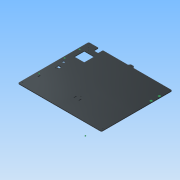
# Autodesk Inventor part: боковая  панель
Saved by Autodesk Inventor 2017 (Build 210142000, 142)
## iProperties
Part Number: боковая  панель
Material: Типовые
Document SubType Name: Modeling
Designer: Max
Mass: 347.039 g
Surface Area: 2371.89 cm^2
Volume: 347.039 cm^3
Density: 1 g/cm^3
Appearance: Чугун серый
Author: Max
Autodesk Inventor part; units mm, degrees
ref_plane "YZ Plane" through (0, 0, 0) normal (1, 0, 0) x (0, 1, 0)
ref_plane "XZ Plane" through (0, 0, 0) normal (0, 1, 0) x (-1, 0, 0)
ref_plane "XY Plane" through (0, 0, 0) normal (0, 0, 1) x (1, 0, 0)
sketch "Эскиз1" plane through (0, 0, 0) normal (0, 0, 1) x (1, 0, 0)
  circle A0 centre (10.6994, 67.6713) radius 1.5
  circle A1 centre (10.6994, 364.6713) radius 1.5
  circle A2 centre (-348.3006, 364.6713) radius 1.5
  circle A3 centre (-348.3006, 67.6713) radius 1.5
  line L0 (-355.8006, 370.6713) -> (18.1994, 370.6713)
  line L1 (18.1994, 370.6713) -> (18.1994, 53.6713)
  line L2 (18.1994, 53.6713) -> (-355.8006, 53.6713)
  line L3 (-355.8006, 53.6713) -> (-355.8006, 370.6713)
  point P0 (18.1994, 53.6713)
  dimension "d4" = 374
  dimension "d6" = 317
  dimension "d7" = 14
  dimension "d40" = 7.5
  dimension "d41" = 297
  dimension "d42" = 7.5
  dimension "d43" = 7.5
  dimension "d44" = 297
  dimension "d45" = 6
  dimension "d46" = 359
  dimension "d47" = 14
  dimension "d48" = 359
  constraints: 8 end point, 4 centre point, 2 parallel, 1 coincident, 1 horizontal, 1 perpendicular
  measures "d4" distance between parallel lines of L1 L3
  measures "d6" distance between parallel lines of L0 L2
  measures "d7" distance from line of A3.centre L2
  measures "d40" distance from line of L1 A0.centre
  measures "d41" distance of A0.centre A1.centre
  measures "d42" distance from line of L1 A1.centre
  measures "d43" distance from line of L3 A2.centre
  measures "d44" distance of A3.centre A2.centre
  measures "d45" distance from line of L0 A2.centre
  measures "d46" distance of A0.centre A3.centre
  measures "d47" distance from line of L2 A0.centre
  measures "d48" distance of A1.centre A2.centre
extrude "Выдавливание1" add sketch "Эскиз1" along normal blind 3
sketch "Эскиз3" plane through (0, 0, 3) normal (0, 0, 1) x (1, 0, 0)
  circle A0 centre (10.6994, 282.6713) radius 3.75 projected
  circle A1 centre (10.6994, 319.6713) radius 3.75 projected
  circle A2 centre (-348.3006, 321.6713) radius 2 projected
  circle A3 centre (-348.3006, 254.6713) radius 2 projected
  circle A4 centre (-345.3006, 137.6713) radius 1.5 projected
  point P0 (0, 0)
sketch "Эскиз4" plane through (0, 0, 3) normal (0, 0, 1) x (1, 0, 0)
  circle A0 centre (-168.3006, 372.6713) radius 1.5 projected
  line L0 (-179.3006, 370.6713) -> (-175.8006, 378.6713)
  line L1 (-175.8006, 378.6713) -> (-160.8006, 378.6713)
  line L2 (-160.8006, 378.6713) -> (-157.3006, 370.6713)
  line L3 (18.1994, 370.6713) -> (-355.8006, 370.6713) projected
  line L4 (-168.3006, 372.6713) -> (-168.3006, 378.6713)
  point P0 (0, 0)
  dimension "d49" = 8
  dimension "d50" = 22
  dimension "d51" = 15
  constraints: 8 end point, 2 point on line, 1 horizontal, 1 midpoint, 1 perpendicular, 1 other
  measures "d49" distance between parallel lines of L3 L1
  measures "d50" distance of L0.start L2.end
  measures "d51" distance of L0.end L1.end
extrude "Выдавливание3" add sketch "Эскиз4" against normal blind 3
fillet "Сопряжение1" radius 5 4 edges at (-179.3006, 370.6713, 1.5) (-157.3006, 370.6713, 1.5) (-160.8006, 378.6713, 1.5) (-175.8006, 378.6713, 1.5)
fillet "Сопряжение2" radius 5 4 edges at (-355.8006, 370.6713, 1.5) (18.1994, 370.6713, 1.5) (18.1994, 53.6713, 1.5) (-355.8006, 53.6713, 1.5)
sketch "Эскиз5" plane through (0, 0, 3) normal (0, 0, 1) x (1, 0, 0)
  line L0 (-332.3006, 327.1713) -> (-287.3006, 327.1713)
  line L1 (-287.3006, 327.1713) -> (-287.3006, 282.1713)
  line L2 (-287.3006, 282.1713) -> (-332.3006, 282.1713)
  line L3 (-332.3006, 282.1713) -> (-332.3006, 327.1713)
  line L4 (-355.8006, 365.6713) -> (-355.8006, 58.6713) projected
  line L5 (-182.5707, 370.6713) -> (-350.8006, 370.6713) projected
  line L6 (-312.3006, 370.6713) -> (-292.3006, 370.6713)
  line L7 (-292.3006, 370.6713) -> (-292.3006, 349.1713)
  line L8 (-292.3006, 349.1713) -> (-312.3006, 349.1713)
  line L9 (-312.3006, 349.1713) -> (-312.3006, 370.6713)
  circle A0 centre (-335.8006, 238.6713) radius 4.95
  line L10 (-333.3006, 213.1713) -> (-320.3006, 213.1713)
  line L11 (-320.3006, 213.1713) -> (-320.3006, 203.1713)
  line L12 (-320.3006, 203.1713) -> (-333.3006, 203.1713)
  line L13 (-333.3006, 203.1713) -> (-333.3006, 213.1713)
  circle A1 centre (-330.4506, 196.6713) radius 1.6
  circle A2 centre (-323.1506, 196.6713) radius 1.6
  line L14 (-330.4506, 196.6713) -> (-323.1506, 196.6713)
  line L15 (-326.8006, 203.1713) -> (-326.8006, 196.6713)
  circle A3 centre (-162.8006, 142.6713) radius 1.6
  line L16 (18.1994, 58.6713) -> (18.1994, 365.6713) projected
  line L17 (-350.8006, 53.6713) -> (13.1994, 53.6713) projected
  line L18 (-173.8006, 132.1713) -> (-173.8006, 123.1713) construction
  line L19 (-175.3006, 132.1713) -> (-175.3006, 123.1713)
  line L20 (-172.3006, 123.1713) -> (-172.3006, 132.1713)
  arc A4 (-172.3006, 132.1713) -> (-175.3006, 132.1713) centre (-173.8006, 132.1713) ccw
  arc A5 (-175.3006, 123.1713) -> (-172.3006, 123.1713) centre (-173.8006, 123.1713) ccw
  line L21 (-151.8006, 132.1713) -> (-151.8006, 123.1713) construction
  line L22 (-153.3006, 132.1713) -> (-153.3006, 123.1713)
  line L23 (-150.3006, 123.1713) -> (-150.3006, 132.1713)
  arc A6 (-150.3006, 132.1713) -> (-153.3006, 132.1713) centre (-151.8006, 132.1713) ccw
  arc A7 (-153.3006, 123.1713) -> (-150.3006, 123.1713) centre (-151.8006, 123.1713) ccw
  line L24 (-162.8006, 142.6713) -> (-162.8006, 102.5696) construction
  line L25 (-173.8006, 127.6713) -> (-151.8006, 127.6713) construction
  circle A8 centre (-346.3006, 134.6713) radius 1.6
  line L26 (-335.3006, 132.1713) -> (-335.3006, 123.1713)
  line L27 (-336.8006, 132.1713) -> (-336.8006, 123.1713)
  line L28 (-333.8006, 123.1713) -> (-333.8006, 132.1713)
  arc A9 (-333.8006, 132.1713) -> (-336.8006, 132.1713) centre (-335.3006, 132.1713) ccw
  arc A10 (-336.8006, 123.1713) -> (-333.8006, 123.1713) centre (-335.3006, 123.1713) ccw
  circle A11 centre (-334.3006, 349.1713) radius 1.45
  circle A12 centre (-325.3006, 338.6713) radius 1.45
  circle A13 centre (10.6994, 319.6713) radius 3.75 construction
  circle A14 centre (10.6994, 282.6713) radius 3.75 construction
  circle A15 centre (10.6994, 319.6713) radius 4.75
  circle A16 centre (10.6994, 282.6713) radius 4.75
  point P0 (0, 0)
  point P1 (-335.3006, 127.6713)
  dimension "d56" = 68.5
  dimension "d57" = 45
  dimension "d58" = 45
  dimension "d59" = 23.5
  dimension "d60" = 43.5
  dimension "d61" = 21.5
  dimension "d62" = 20
  dimension "d63" = 43.5
  dimension "d64" = 20
  dimension "d65" = 132
  dimension "d66" = 9.9
  dimension "d67" = 13
  dimension "d68" = 10
  dimension "d69" = 157.5
  dimension "d70" = 22.5
  dimension "d71" = 3.2
  dimension "d72" = 3.2
  dimension "d73" = 10.5
  dimension "d74" = 6.5
  dimension "d75" = 7.3
  dimension "d76" = 193
  dimension "d77" = 181
  dimension "d78" = 89
  dimension "d79" = 3.2
  dimension "d80" = 22
  dimension "d81" = 12
  dimension "d82" = 3
  dimension "d83" = 3
  dimension "d84" = 12
  dimension "d85" = 25
  dimension "d86" = 68
  dimension "d87" = 3.2
  dimension "d88" = 9.5
  dimension "d89" = 81
  dimension "d90" = 3
  dimension "d91" = 68
  dimension "d92" = 19
  dimension "d93" = 12
  dimension "d94" = 2.9
  dimension "d95" = 2.9
  dimension "d96" = 21.5
  dimension "d97" = 21.5
  dimension "d98" = 32
  dimension "d99" = 30.5
  dimension "d100" = 9.5
  dimension "d101" = 9.5
  constraints: 56 end point, 15 centre point, 12 point on circle, 12 tangent, 10 parallel, 5 horizontal, 5 midpoint, 4 perpendicular, 3 coincident, 3 vertical, 1 point on line, 1 symmetric about line, 1 other
  measures "d56" distance between parallel lines of L1 L4
  measures "d57" distance between parallel lines of L2 L0
  measures "d58" distance between parallel lines of L1 L3
  measures "d59" distance between parallel lines of L3 L4
  measures "d60" distance between parallel lines of L0 L5
  measures "d61" distance between parallel lines of L8 L5
  measures "d62" distance between parallel lines of L7 L9
  measures "d63" distance between parallel lines of L9 L4
  measures "d64" distance from line of L4 A0.centre
  measures "d65" distance from line of L5 A0.centre
  measures "d66" diameter of A0
  measures "d67" distance of L11.end L12.end
  measures "d68" distance of L10.end L11.end
  measures "d69" distance between parallel lines of L5 L10
  measures "d70" distance between parallel lines of L4 L13
  measures "d71" diameter of A2
  measures "d72" diameter of A1
  measures "d74" distance from line of L12 L14.start
  measures "d75" distance of L14.end L14.start
  measures "d76" distance from line of L4 L24.start
  measures "d77" distance from line of L16 L24.start
  measures "d78" distance from line of L17 L24.start
  measures "d79" diameter of A3
  measures "d80" distance between parallel lines of L21 L18
  measures "d82" distance between parallel lines of L20 L19
  measures "d83" distance between parallel lines of L23 L22
  measures "d85" distance between parallel lines of L23 L19
  measures "d86" distance edge to line of A5 L17
  measures "d87" diameter of A8
  measures "d88" distance from line of L4 A8.centre
  measures "d89" distance from line of L17 A8.centre
  measures "d90" diameter of A10
  measures "d91" distance edge to line of A10 L17
  measures "d92" distance between parallel lines of L4 L27
  measures "d94" diameter of A11
  measures "d95" diameter of A12
  measures "d96" distance from line of A11.centre L5
  measures "d97" distance from line of L4 A11.centre
  measures "d98" distance from line of L5 A12.centre
  measures "d99" distance from line of L4 A12.centre
  measures "d100" diameter of A15
  measures "d101" diameter of A16
extrude "Выдавливание4" cut sketch "Эскиз5" against normal blind 10
fillet "Сопряжение3" radius 2 12 edges at (-312.3006, 370.6713, 1.5) (-292.3006, 370.6713, 1.5) (-312.3006, 349.1713, 1.5) (-292.3006, 349.1713, 1.5) (-332.3006, 327.1713, 1.5) (-287.3006, 327.1713, 1.5) (-287.3006, 282.1713, 1.5) (-332.3006, 282.1713, 1.5) (-333.3006, 203.1713, 1.5) (-333.3006, 213.1713, 1.5) (-320.3006, 213.1713, 1.5) (-320.3006, 203.1713, 1.5)
sketch "Эскиз6" plane through (0, 0, 3) normal (0, 0, 1) x (1, 0, 0)
  circle A0 centre (-348.3006, 335.6713) radius 2 projected
  circle A1 centre (-348.3006, 282.6713) radius 2 projected
  circle A2 centre (-348.3006, 254.6713) radius 2 projected
  circle A3 centre (-348.3006, 321.6713) radius 2 projected
  line L0 (-359.8006, 317.6713) -> (-359.8006, 321.6713) projected
  point P0 (0, 0)
  dimension "d107" = 67
  measures "d107" distance of A2.centre A3.centre
extrude "Выдавливание5" cut sketch "Эскиз6" against normal blind 10 contours A2 | A3
